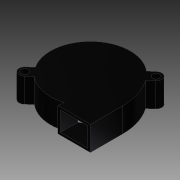
# Autodesk Inventor part: fan
Saved by Autodesk Inventor 2013 (Build 170138000, 138)
## iProperties
Created: 2014-10-26
Part Number: fan
Material: Acetal Resin, Black
Document SubType Name: Modeling
Designer: Masta
Density: 1 g/cm^3
Author: Masta
Autodesk Inventor part; units mm, degrees
ref_plane "YZ Plane" through (0, 0, 0) normal (1, 0, 0) x (0, 1, 0)
ref_plane "XZ Plane" through (0, 0, 0) normal (0, 1, 0) x (-1, 0, 0)
ref_plane "XY Plane" through (0, 0, 0) normal (0, 0, 1) x (1, 0, 0)
sketch "Sketch1" plane through (0, 0, 0) normal (0, 0, 1) x (1, 0, 0)
  arc A0 (18.957, 15.5204) -> (15.8526, 18.6801) centre (0, 0) ccw construction
  line L0 (-24.5, 24.5) -> (27, 24.5) construction
  line L1 (27, 24.5) -> (27, -27) construction
  line L2 (27, -27) -> (-24.5, -27) construction
  line L3 (-24.5, -27) -> (-24.5, 24.5) construction
  line L4 (7, -27) -> (27, -27)
  line L5 (27, -27) -> (27, -7)
  arc A1 (27, -7) -> (20.52, 13.4631) centre (-8.55, -7) ccw
  line L6 (7, -27) -> (7, -23.4787)
  line L7 (21.5, 19) -> (0, 0) construction
  line L8 (-21.5, -19) -> (0, 0) construction
  arc A2 (18.8773, 16.6823) -> (23.8177, 16.3773) centre (21.5, 19) ccw construction
  arc A3 (-23.8177, -16.3773) -> (-19.1823, -21.6227) centre (-21.5, -19) ccw
  line L9 (-23.8177, -16.3773) -> (-20.488, -13.4348)
  line L10 (-19.1823, -21.6227) -> (-15.8526, -18.6801)
  line L11 (23.8177, 16.3773) -> (20.52, 13.4631)
  line L12 (19.1823, 21.6227) -> (15.8526, 18.6801)
  arc A4 (7, -23.4787) -> (18.957, 15.5204) centre (0, 0) ccw construction
  arc A5 (15.8526, 18.6801) -> (-20.488, -13.4348) centre (0, 0) ccw
  arc A6 (20.52, 13.4631) -> (18.957, 15.5204) centre (-8.55, -7) ccw construction
  arc A7 (19.1823, 21.6227) -> (18.8773, 16.6823) centre (21.5, 19) ccw construction
  arc A8 (23.8177, 16.3773) -> (19.1823, 21.6227) centre (21.5, 19) ccw
  arc A9 (-18.8773, -16.6823) -> (-23.8177, -16.3773) centre (-21.5, -19) ccw construction
  arc A10 (-19.1823, -21.6227) -> (-18.8773, -16.6823) centre (-21.5, -19) ccw construction
  arc A11 (-15.8526, -18.6801) -> (7, -23.4787) centre (0, 0) ccw
  arc A12 (-20.488, -13.4348) -> (-15.8526, -18.6801) centre (0, 0) ccw construction
  dimension "d0" = 49
  dimension "d1" = 51.5
  dimension "d2" = 51.5
  dimension "d3" = 20
  dimension "d4" = 20
  dimension "d5" = 43
  dimension "d6" = 38
  dimension "d7" = 7
  dimension "d8" = 7
  constraints: 29 point on circle, 26 end point, 19 tangent, 13 centre point, 6 parallel, 4 collinear, 4 point on line, 3 coincident, 1 horizontal, 1 perpendicular
  measures "d0" diameter of A0
  measures "d1" distance of L1.end L2.end
  measures "d2" distance of L0.end L1.end
  measures "d3" distance of L1.end L5.end
  measures "d4" distance of L4.start L1.end
  measures "d5" horizontal distance of L8.start L7.start
  measures "d6" vertical distance of L7.start L8.start
  measures "d7" diameter of A2
  measures "d8" diameter of A3
extrude "Extrusion1" add sketch "Sketch1" against normal blind 15
sketch "Sketch2" plane through (7, -27, 0) normal (0, -1, 0) x (1, 0, 0)
  line L0 (20, 0) -> (0, 0) projected
  line L1 (0, 0) -> (0, -15) projected
  line L2 (20, -15) -> (0, -15) projected
  line L3 (20, 0) -> (20, -15) projected
  line L4 (1.5, -1.5) -> (18.5, -1.5)
  line L5 (18.5, -1.5) -> (18.5, -13.5)
  line L6 (18.5, -13.5) -> (1.5, -13.5)
  line L7 (1.5, -13.5) -> (1.5, -1.5)
  point P0 (-7, 0)
  dimension "d22" = 1.5
  constraints: 8 end point, 3 other
  measures "d22" distance between parallel lines of L0 L4
extrude "Extrusion2" cut sketch "Sketch2" against normal blind 25 contours L4 L5 L6 L7
hole "Hole1" at (-21.5, -19, 0) at (21.5, 19, 0) direction (0, 0, -1) diameter 4.4 end through all
sketch "Sketch3" plane through (0, 0, -15) normal (0, 0, -1) x (-1, 0, 0)
  arc A0 (20.488, -13.4348) -> (-15.8526, 18.6801) centre (0, 0) ccw projected
  circle A1 centre (0, 0) radius 18.3084
  circle A2 centre (0, 0) radius 11.7236
  constraints: 2 centre point, 2 coincident
extrude "Extrusion3" cut sketch "Sketch3" against normal blind 13.5
body "Solid1"
